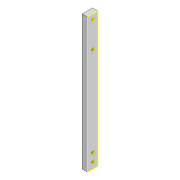
# Autodesk Inventor part: Vertical_bar
Saved by Autodesk Inventor 2022 (Build 260153000, 153)
## iProperties
Created: 2022-08-23
Part Number: Vertical_bar
Material: Generic
Document SubType Name: Modeling
Designer: dell
Density: 1 g/cm^3
Appearance: Default
Mass: 6.42931 g
Surface Area: 40.6597 cm^2
Volume: 6.42931 cm^3
Author: dell
Autodesk Inventor part; units mm, degrees
ref_plane "YZ Plane" through (0, 0, 0) normal (1, 0, 0) x (0, 1, 0)
ref_plane "XZ Plane" through (0, 0, 0) normal (0, 1, 0) x (-1, 0, 0)
ref_plane "XY Plane" through (0, 0, 0) normal (0, 0, 1) x (1, 0, 0)
sketch "Sketch1" plane through (0, 0, 0) normal (1, 0, 0) x (0, 1, 0)
  line L0 (0, 0) -> (130, 0)
  line L1 (130, 0) -> (130, -10)
  line L2 (130, -10) -> (0, -10)
  line L3 (0, -10) -> (0, 0)
  circle A0 centre (125, -5) radius 1.5
  circle A1 centre (100, -5) radius 1.5
  circle A2 centre (14, -5) radius 1.5
  circle A3 centre (6, -5) radius 1.5
  dimension "d0" = 130
  dimension "d1" = 10
  dimension "d4" = 3
  dimension "d5" = 5
  dimension "d6" = 3
  dimension "d8" = 25
  dimension "d15" = 3
  dimension "d16" = 3
  dimension "d17" = 5
  dimension "d18" = 5
  dimension "d19" = 116
  dimension "d20" = 124
  constraints: 8 end point, 4 centre point, 2 parallel, 1 horizontal, 1 perpendicular
  measures "d0" distance of L1.end L2.end
  measures "d1" distance between parallel lines of L0 L2
  measures "d4" diameter of A0
  measures "d5" distance from line of L1 A0.centre
  measures "d6" diameter of A1
  measures "d8" distance of A1.centre A0.centre
  measures "d15" diameter of A2
  measures "d16" diameter of A3
  measures "d17" distance from line of L0 A2.centre
  measures "d18" distance from line of L0 A3.centre
  measures "d19" distance from line of L1 A2.centre
  measures "d20" distance from line of L1 A3.centre
extrude "Extrusion1" add sketch "Sketch1" along normal blind 5
sketch "Sketch3" plane through (5, 0, 0) normal (1, 0, 0) x (0, 0, -1)
  circle A0 centre (5, 125) radius 1.5 projected
  circle A1 centre (5, 100) radius 1.5 projected
  circle A2 centre (5, 14) radius 1.5 projected
  circle A3 centre (5, 6) radius 1.5 projected
  line L0 (10, 0) -> (0, 0) projected
  line L1 (0, 0) -> (0, 130) projected
  line L2 (0, 130) -> (10, 130) projected
  line L3 (10, 130) -> (10, 0) projected
body "Solid1"
